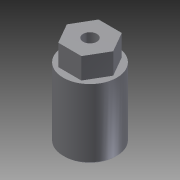
# Autodesk Inventor part: MotorToHexKey
Saved by Autodesk Inventor 2012 (Build 160160000, 160)
## iProperties
Created: 2011-10-18
Part Number: MotorToHexKey
Material: Default
Document SubType Name: Modeling
Designer: KuttaA
Density: 1 g/cm^3
Author: KuttaA
Autodesk Inventor part; units mm, degrees
ref_plane "YZ Plane" through (0, 0, 0) normal (1, 0, 0) x (0, 1, 0)
ref_plane "XZ Plane" through (0, 0, 0) normal (0, 1, 0) x (-1, 0, 0)
ref_plane "XY Plane" through (0, 0, 0) normal (0, 0, 1) x (1, 0, 0)
sketch "Sketch1" plane through (0, 0, 0) normal (0, 0, 1) x (1, 0, 0)
  circle A0 centre (0, 0) radius 8
  dimension "d0" = 16
  constraints: 1 centre point, 1 coincident
  measures "d0" diameter of A0
extrude "Extrusion1" add sketch "Sketch1" along normal blind 20.65
chamfer "Chamfer1" distance 0.5 angle 45 1 edges at (-8, 0, 0)
sketch "Sketch2" plane through (0, 0, 20.65) normal (0, 0, 1) x (1, 0, 0)
  circle A0 centre (0, 0) radius 8 projected
  line L0 (3.4803, 5.9906) -> (6.9282, -0.0187)
  line L1 (6.9282, -0.0187) -> (3.4479, -6.0093)
  line L2 (3.4479, -6.0093) -> (-3.4803, -5.9906)
  line L3 (-3.4803, -5.9906) -> (-6.9282, 0.0187)
  line L4 (-6.9282, 0.0187) -> (-3.4479, 6.0093)
  line L5 (-3.4479, 6.0093) -> (3.4803, 5.9906)
  line L6 (0, 0) -> (3.4803, 5.9906)
  line L7 (0, 0) -> (-3.4479, 6.0093)
  line L8 (-6.9282, 0.0187) -> (0, 0)
  line L9 (-3.4803, -5.9906) -> (0, 0)
  line L10 (3.4479, -6.0093) -> (0, 0)
  line L11 (6.9282, -0.0187) -> (0, 0)
  dimension "d9" = 12
  constraints: 24 end point, 7 equal length, 3 parallel
  measures "d9" distance between parallel lines of L1 L4
extrude "Extrusion2" add sketch "Sketch2" along normal blind 6.3 contours L6 L7 L5 | L0 L11 L6 | L1 L10 L11 | L7 L8 L4 | L9 L3 L8 | L10 L2 L9
sketch "Sketch3" plane through (0, 0, 0) normal (0, 0, -1) x (-1, 0, 0)
  circle A0 centre (0, 0) radius 2.05
  dimension "d10" = 4.1
  constraints: 1 centre point, 1 coincident
  measures "d10" diameter of A0
extrude "Extrusion3" cut sketch "Sketch3" against normal through all
sketch "Sketch4" plane through (0, 0, 0) normal (0, 0, -1) x (-1, 0, 0)
  circle A0 centre (0, 0) radius 3.1
  dimension "d16" = 6.2
  constraints: 1 centre point, 1 coincident
  measures "d16" diameter of A0
extrude "Extrusion4" cut sketch "Sketch4" against normal blind 20
chamfer "Chamfer3" distance 0.5 angle 45 1 edges at (3.1, 0, 0)
sketch "Sketch5" plane through (0, 0, 0) normal (1, 0, 0) x (0, 1, 0)
  circle A0 centre (0, 6.5) radius 2.4
  line L0 (7.5, 0) -> (-7.5, 0) projected
  line L1 (-3.6, 0) -> (3.6, 0) projected
  point P0 (0, 0)
  dimension "d22" = 4.8
  dimension "d23" = 6.5
  constraints: 1 centre point
  measures "d22" diameter of A0
  measures "d23" distance from line of L0 A0.centre
extrude "Extrusion5" cut sketch "Sketch5" against normal blind 10
body "Solid1"
